Autodesk Fusion 360 part; units mm, degrees
(part 2 of 2)
sketch "Sketch5" plane through (0, 0, -2) normal (0, 0, -1) x (1, 0, 0)
  circle A0 centre (59.3355, -41.7346) radius 3
  circle A1 centre (58.8128, 16.7193) radius 3
  circle A2 centre (6.5755, -41.7346) radius 3
  circle A3 centre (6.5514, 16.7159) radius 3
  arc A4 (0, -61.8304) -> (1, -62.8304) centre (1, -61.8304) ccw
  line L0 (1, -62.8304) -> (64.3008, -62.8304)
  arc A5 (64.3008, -62.8304) -> (65.3008, -61.8304) centre (64.3008, -61.8304) ccw
  line L1 (65.3008, -61.8304) -> (65.3008, 30)
  line L2 (65.3008, 30) -> (55.2691, 40)
  line L3 (55.2691, 40) -> (10, 40)
  line L4 (10, 40) -> (0, 30)
  line L5 (0, 30) -> (0, -61.8304)
  line L6 (49.6443, -61.9222) -> (53.0574, -58.8103)
  line L7 (39.6674, -44.8986) -> (36.2543, -48.0106)
  line L8 (36.2543, -40.0106) -> (37.2428, -44.5224)
  line L9 (61.0574, -18.8103) -> (60.0689, -14.2985)
  line L10 (52.2543, -56.0106) -> (53.2428, -60.5224)
  line L11 (61.0574, -50.8103) -> (60.0689, -46.2985)
  line L12 (55.6674, -44.8986) -> (52.2543, -48.0106)
  line L13 (53.0574, -58.8103) -> (52.0689, -54.2985)
  line L14 (39.6674, -12.8986) -> (36.2543, -16.0106)
  line L15 (52.2543, -16.0106) -> (53.2428, -20.5224)
  line L16 (53.2428, -20.5224) -> (57.6443, -21.9222)
  line L17 (53.2428, -28.5224) -> (57.6443, -29.9222)
  line L18 (53.0574, -34.8103) -> (52.0689, -30.2985)
  line L19 (61.0574, -26.8103) -> (60.0689, -22.2985)
  line L20 (52.2543, -24.0106) -> (53.2428, -28.5224)
  line L21 (52.2543, -32.0106) -> (53.2428, -36.5224)
  line L22 (61.0574, -34.8103) -> (60.0689, -30.2985)
  line L23 (60.0689, -30.2985) -> (55.6674, -28.8986)
  line L24 (49.6443, -29.9222) -> (53.0574, -26.8103)
  line L25 (55.6674, -28.8986) -> (52.2543, -32.0106)
  line L26 (57.6443, -29.9222) -> (61.0574, -26.8103)
  line L27 (49.6443, -21.9222) -> (53.0574, -18.8103)
  line L28 (53.0574, -26.8103) -> (52.0689, -22.2985)
  line L29 (60.0689, -38.2985) -> (55.6674, -36.8986)
  line L30 (45.2428, -28.5224) -> (49.6443, -29.9222)
  line L31 (39.6674, -28.8986) -> (36.2543, -32.0106)
  line L32 (45.0574, -26.8103) -> (44.0689, -22.2985)
  line L33 (33.6443, -37.9222) -> (37.0574, -34.8103)
  line L34 (44.2543, -16.0106) -> (45.2428, -20.5224)
  line L35 (37.2428, -36.5224) -> (41.6443, -37.9222)
  line L36 (44.2543, -24.0106) -> (45.2428, -28.5224)
  line L37 (44.2543, -32.0106) -> (45.2428, -36.5224)
  line L38 (41.6443, -37.9222) -> (45.0574, -34.8103)
  line L39 (37.0574, -26.8103) -> (36.0689, -22.2985)
  line L40 (44.0689, -30.2985) -> (39.6674, -28.8986)
  line L41 (52.0689, -46.2985) -> (47.6674, -44.8986)
  line L42 (45.2428, -52.5224) -> (49.6443, -53.9222)
  line L43 (61.0574, -58.8103) -> (60.0689, -54.2985)
  line L44 (45.2428, -44.5224) -> (49.6443, -45.9222)
  line L45 (52.0689, -54.2985) -> (47.6674, -52.8986)
  line L46 (53.2428, -52.5224) -> (57.6443, -53.9222)
  line L47 (36.2543, -16.0106) -> (37.2428, -20.5224)
  line L48 (45.2428, -60.5224) -> (49.6443, -61.9222)
  line L49 (53.2428, -60.5224) -> (57.6443, -61.9222)
  line L50 (60.0689, -46.2985) -> (55.6674, -44.8986)
  line L51 (55.6674, -52.8986) -> (52.2543, -56.0106)
  line L52 (60.0689, -54.2985) -> (55.6674, -52.8986)
  line L53 (49.6443, -53.9222) -> (53.0574, -50.8103)
  line L54 (47.6674, -28.8986) -> (44.2543, -32.0106)
  line L55 (41.6443, -29.9222) -> (45.0574, -26.8103)
  line L56 (33.6443, -29.9222) -> (37.0574, -26.8103)
  line L57 (49.6443, -37.9222) -> (53.0574, -34.8103)
  line L58 (57.6443, -21.9222) -> (61.0574, -18.8103)
  line L59 (57.6443, -37.9222) -> (61.0574, -34.8103)
  line L60 (60.0689, -22.2985) -> (55.6674, -20.8986)
  line L61 (55.6674, -20.8986) -> (52.2543, -24.0106)
  line L62 (53.2428, -36.5224) -> (57.6443, -37.9222)
  line L63 (44.0689, -38.2985) -> (39.6674, -36.8986)
  line L64 (45.0574, -34.8103) -> (44.0689, -30.2985)
  line L65 (47.6674, -20.8986) -> (44.2543, -24.0106)
  line L66 (39.6674, -20.8986) -> (36.2543, -24.0106)
  line L67 (33.6443, -21.9222) -> (37.0574, -18.8103)
  line L68 (36.2543, -24.0106) -> (37.2428, -28.5224)
  line L69 (37.2428, -28.5224) -> (41.6443, -29.9222)
  line L70 (37.2428, -20.5224) -> (41.6443, -21.9222)
  line L71 (41.6443, -21.9222) -> (45.0574, -18.8103)
  line L72 (44.0689, -22.2985) -> (39.6674, -20.8986)
  line L73 (36.2543, -32.0106) -> (37.2428, -36.5224)
  line L74 (37.0574, -34.8103) -> (36.0689, -30.2985)
  line L75 (37.2428, -12.5224) -> (41.6443, -13.9222)
  line L76 (29.2428, -36.5224) -> (33.6443, -37.9222)
  line L77 (31.6674, -28.8986) -> (28.2543, -32.0106)
  line L78 (61.0574, 5.1897) -> (60.0689, 9.7015)
  line L79 (44.2543, -8.0106) -> (45.2428, -12.5224)
  line L80 (33.6443, 18.0778) -> (37.0574, 21.1897)
  line L81 (55.6674, 11.1014) -> (52.2543, 7.9894)
  line L82 (36.0689, -54.2985) -> (31.6674, -52.8986)
  line L83 (33.6443, 26.0778) -> (37.0574, 29.1897)
  line L84 (47.6674, -4.8986) -> (44.2543, -8.0106)
  line L85 (44.0689, -6.2985) -> (39.6674, -4.8986)
  line L86 (37.0574, 5.1897) -> (36.0689, 9.7015)
  line L87 (21.2428, -20.5224) -> (25.6443, -21.9222)
  line L88 (29.2428, -44.5224) -> (33.6443, -45.9222)
  line L89 (44.2543, -0.0106) -> (45.2428, -4.5224)
  line L90 (33.6443, -5.9222) -> (37.0574, -2.8103)
  line L91 (15.6674, 11.1014) -> (12.2543, 7.9894)
  line L92 (37.2428, 3.4776) -> (41.6443, 2.0778)
  line L93 (36.0689, 25.7015) -> (31.6674, 27.1014)
  line L94 (44.2543, 7.9894) -> (45.2428, 3.4776)
  line L95 (29.2428, -60.5224) -> (33.6443, -61.9222)
  line L96 (41.6443, -13.9222) -> (45.0574, -10.8103)
  line L97 (36.2543, 7.9894) -> (37.2428, 3.4776)
  line L98 (36.0689, -46.2985) -> (31.6674, -44.8986)
  line L99 (37.2428, -4.5224) -> (41.6443, -5.9222)
  line L100 (13.0574, 5.1897) -> (12.0689, 9.7015)
  line L101 (44.0689, -14.2985) -> (39.6674, -12.8986)
  line L102 (39.6674, 3.1014) -> (36.2543, -0.0106)
  line L103 (45.0574, -2.8103) -> (44.0689, 1.7015)
  line L104 (28.0689, -30.2985) -> (23.6674, -28.8986)
  line L105 (31.6674, 11.1014) -> (28.2543, 7.9894)
  line L106 (28.2543, -16.0106) -> (29.2428, -20.5224)
  line L107 (15.6674, -36.8986) -> (12.2543, -40.0106)
  line L108 (25.6443, -29.9222) -> (29.0574, -26.8103)
  line L109 (57.6443, 2.0778) -> (61.0574, 5.1897)
  line L110 (28.2543, -8.0106) -> (29.2428, -12.5224)
  line L111 (13.0574, -42.8103) -> (12.0689, -38.2985)
  line L112 (31.6674, 3.1014) -> (28.2543, -0.0106)
  line L113 (28.0689, -22.2985) -> (23.6674, -20.8986)
  line L114 (47.6674, 11.1014) -> (44.2543, 7.9894)
  line L115 (57.6443, -13.9222) -> (61.0574, -10.8103)
  line L116 (25.6443, -13.9222) -> (29.0574, -10.8103)
  line L117 (31.6674, -20.8986) -> (28.2543, -24.0106)
  line L118 (29.0574, -34.8103) -> (28.0689, -30.2985)
  line L119 (23.6674, -36.8986) -> (20.2543, -40.0106)
  line L120 (21.0574, -26.8103) -> (20.0689, -22.2985)
  line L121 (53.0574, -2.8103) -> (52.0689, 1.7015)
  line L122 (17.6443, -29.9222) -> (21.0574, -26.8103)
  line L123 (20.2543, -32.0106) -> (21.2428, -36.5224)
  line L124 (29.2428, 3.4776) -> (33.6443, 2.0778)
  line L125 (20.2543, 7.9894) -> (21.2428, 3.4776)
  line L126 (21.2428, -12.5224) -> (25.6443, -13.9222)
  line L127 (17.6443, -21.9222) -> (21.0574, -18.8103)
  line L128 (39.6674, 11.1014) -> (36.2543, 7.9894)
  line L129 (29.0574, -26.8103) -> (28.0689, -22.2985)
  line L130 (36.0689, -22.2985) -> (31.6674, -20.8986)
  line L131 (29.2428, -4.5224) -> (33.6443, -5.9222)
  line L132 (29.0574, 5.1897) -> (28.0689, 9.7015)
  line L133 (28.2543, -24.0106) -> (29.2428, -28.5224)
  line L134 (53.2428, -12.5224) -> (57.6443, -13.9222)
  line L135 (23.6674, 11.1014) -> (20.2543, 7.9894)
  line L136 (49.6443, -13.9222) -> (53.0574, -10.8103)
  line L137 (9.6443, -45.9222) -> (13.0574, -42.8103)
  line L138 (29.2428, -28.5224) -> (33.6443, -29.9222)
  line L139 (5.2428, -60.5224) -> (9.6443, -61.9222)
  line L140 (9.6443, -53.9222) -> (13.0574, -50.8103)
  line L141 (37.0574, -10.8103) -> (36.0689, -6.2985)
  line L142 (5.2428, -52.5224) -> (9.6443, -53.9222)
  line L143 (12.2543, -48.0106) -> (13.2428, -52.5224)
  line L144 (36.0689, -30.2985) -> (31.6674, -28.8986)
  line L145 (36.2543, -8.0106) -> (37.2428, -12.5224)
  line L146 (36.0689, 9.7015) -> (31.6674, 11.1014)
  line L147 (4.2543, -48.0106) -> (5.2428, -52.5224)
  line L148 (12.0689, -54.2985) -> (7.6674, -52.8986)
  line L149 (4.2543, -56.0106) -> (5.2428, -60.5224)
  line L150 (36.0689, -38.2985) -> (31.6674, -36.8986)
  line L151 (33.6443, 10.0778) -> (37.0574, 13.1897)
  line L152 (36.0689, -14.2985) -> (31.6674, -12.8986)
  line L153 (13.2428, -60.5224) -> (17.6443, -61.9222)
  line L154 (15.6674, -44.8986) -> (12.2543, -48.0106)
  line L155 (29.2428, -52.5224) -> (33.6443, -53.9222)
  line L156 (7.6674, -44.8986) -> (4.2543, -48.0106)
  line L157 (5.2428, -44.5224) -> (9.6443, -45.9222)
  line L158 (36.0689, -6.2985) -> (31.6674, -4.8986)
  line L159 (41.6443, 2.0778) -> (45.0574, 5.1897)
  line L160 (45.0574, -10.8103) -> (44.0689, -6.2985)
  line L161 (29.2428, -20.5224) -> (33.6443, -21.9222)
  line L162 (41.6443, -5.9222) -> (45.0574, -2.8103)
  line L163 (36.0689, 17.7015) -> (31.6674, 19.1014)
  line L164 (44.0689, 1.7015) -> (39.6674, 3.1014)
  line L165 (39.6674, -4.8986) -> (36.2543, -8.0106)
  line L166 (20.0689, -46.2985) -> (15.6674, -44.8986)
  line L167 (36.0689, 1.7015) -> (31.6674, 3.1014)
  line L168 (13.2428, -44.5224) -> (17.6443, -45.9222)
  line L169 (33.6443, -13.9222) -> (37.0574, -10.8103)
  line L170 (36.2543, -0.0106) -> (37.2428, -4.5224)
  line L171 (36.0689, 33.7015) -> (31.6674, 35.1014)
  line L172 (13.2428, -52.5224) -> (17.6443, -53.9222)
  line L173 (37.0574, -2.8103) -> (36.0689, 1.7015)
  line L174 (20.0689, -54.2985) -> (15.6674, -52.8986)
  line L175 (33.6443, 2.0778) -> (37.0574, 5.1897)
  line L176 (47.6674, 3.1014) -> (44.2543, -0.0106)
  line L177 (52.0689, -38.2985) -> (47.6674, -36.8986)
  line L178 (45.0574, -42.8103) -> (44.0689, -38.2985)
  line L179 (45.2428, -20.5224) -> (49.6443, -21.9222)
  line L180 (53.0574, -42.8103) -> (52.0689, -38.2985)
  line L181 (52.0689, -30.2985) -> (47.6674, -28.8986)
  line L182 (45.2428, -36.5224) -> (49.6443, -37.9222)
  line L183 (52.0689, -22.2985) -> (47.6674, -20.8986)
  line L184 (47.6674, -36.8986) -> (44.2543, -40.0106)
  line L185 (39.6674, -36.8986) -> (36.2543, -40.0106)
  line L186 (55.6674, -36.8986) -> (52.2543, -40.0106)
  line L187 (61.0574, -42.8103) -> (60.0689, -38.2985)
  line L188 (37.0574, -42.8103) -> (36.0689, -38.2985)
  line L189 (12.2543, -56.0106) -> (13.2428, -60.5224)
  line L190 (12.0689, -46.2985) -> (7.6674, -44.8986)
  line L191 (4.2543, -40.0106) -> (5.2428, -44.5224)
  line L192 (7.6674, -52.8986) -> (4.2543, -56.0106)
  line L193 (23.6674, -12.8986) -> (20.2543, -16.0106)
  line L194 (55.6674, -12.8986) -> (52.2543, -16.0106)
  line L195 (53.0574, -18.8103) -> (52.0689, -14.2985)
  line L196 (7.6674, -12.8986) -> (4.2543, -16.0106)
  line L197 (15.6674, -12.8986) -> (12.2543, -16.0106)
  line L198 (9.6443, -61.9222) -> (13.0574, -58.8103)
  line L199 (13.0574, -58.8103) -> (12.0689, -54.2985)
  line L200 (45.0574, -18.8103) -> (44.0689, -14.2985)
  line L201 (15.6674, -52.8986) -> (12.2543, -56.0106)
  line L202 (12.2543, -40.0106) -> (13.2428, -44.5224)
  line L203 (4.2543, -32.0106) -> (5.2428, -36.5224)
  line L204 (17.6443, -13.9222) -> (21.0574, -10.8103)
  line L205 (4.2543, -16.0106) -> (5.2428, -20.5224)
  line L206 (12.2543, -16.0106) -> (13.2428, -20.5224)
  line L207 (4.2543, -24.0106) -> (5.2428, -28.5224)
  line L208 (39.6674, 35.1014) -> (36.2543, 31.9894)
  line L209 (15.6674, -20.8986) -> (12.2543, -24.0106)
  line L210 (23.6674, -4.8986) -> (20.2543, -8.0106)
  line L211 (29.0574, -10.8103) -> (28.0689, -6.2985)
  line L212 (45.2428, -12.5224) -> (49.6443, -13.9222)
  line L213 (9.6443, -29.9222) -> (13.0574, -26.8103)
  line L214 (45.2428, -4.5224) -> (49.6443, -5.9222)
  line L215 (45.2428, 3.4776) -> (49.6443, 2.0778)
  line L216 (52.0689, -6.2985) -> (47.6674, -4.8986)
  line L217 (41.6443, 10.0778) -> (45.0574, 13.1897)
  line L218 (12.2543, -32.0106) -> (13.2428, -36.5224)
  line L219 (21.0574, -10.8103) -> (20.0689, -6.2985)
  line L220 (37.0574, 29.1897) -> (36.0689, 33.7015)
  line L221 (44.0689, 9.7015) -> (39.6674, 11.1014)
  line L222 (60.0689, -14.2985) -> (55.6674, -12.8986)
  line L223 (20.2543, -8.0106) -> (21.2428, -12.5224)
  line L224 (44.2543, 15.9894) -> (45.2428, 11.4776)
  line L225 (21.2428, -4.5224) -> (25.6443, -5.9222)
  line L226 (52.0689, 1.7015) -> (47.6674, 3.1014)
  line L227 (45.0574, 13.1897) -> (44.0689, 17.7015)
  line L228 (47.6674, 19.1014) -> (44.2543, 15.9894)
  line L229 (52.0689, -14.2985) -> (47.6674, -12.8986)
  line L230 (37.0574, 13.1897) -> (36.0689, 17.7015)
  line L231 (12.0689, -22.2985) -> (7.6674, -20.8986)
  line L232 (52.0689, 17.7015) -> (47.6674, 19.1014)
  line L233 (45.2428, 19.4776) -> (49.6443, 18.0778)
  line L234 (5.2428, 3.4776) -> (9.6443, 2.0778)
  line L235 (29.0574, -42.8103) -> (28.0689, -38.2985)
  line L236 (9.6443, -37.9222) -> (13.0574, -34.8103)
  line L237 (12.2543, 7.9894) -> (13.2428, 3.4776)
  line L238 (9.6443, -21.9222) -> (13.0574, -18.8103)
  line L239 (45.2428, 27.4776) -> (49.6443, 26.0778)
  line L240 (12.0689, 1.7015) -> (7.6674, 3.1014)
  line L241 (12.0689, -6.2985) -> (7.6674, -4.8986)
  line L242 (47.6674, 35.1014) -> (44.2543, 31.9894)
  line L243 (31.6674, -36.8986) -> (28.2543, -40.0106)
  line L244 (12.0689, -38.2985) -> (7.6674, -36.8986)
  line L245 (44.0689, 25.7015) -> (39.6674, 27.1014)
  line L246 (13.0574, -26.8103) -> (12.0689, -22.2985)
  line L247 (7.6674, -28.8986) -> (4.2543, -32.0106)
  line L248 (5.2428, -20.5224) -> (9.6443, -21.9222)
  line L249 (4.2543, -0.0106) -> (5.2428, -4.5224)
  line L250 (44.0689, 33.7015) -> (39.6674, 35.1014)
  line L251 (52.0689, 25.7015) -> (47.6674, 27.1014)
  line L252 (39.6674, 27.1014) -> (36.2543, 23.9894)
  line L253 (4.2543, -8.0106) -> (5.2428, -12.5224)
  line L254 (20.0689, -38.2985) -> (15.6674, -36.8986)
  line L255 (44.2543, 31.9894) -> (45.2428, 27.4776)
  line L256 (12.2543, -24.0106) -> (13.2428, -28.5224)
  line L257 (5.2428, -28.5224) -> (9.6443, -29.9222)
  line L258 (45.0574, 21.1897) -> (44.0689, 25.7015)
  line L259 (13.2428, -28.5224) -> (17.6443, -29.9222)
  line L260 (41.6443, 26.0778) -> (45.0574, 29.1897)
  line L261 (13.0574, -10.8103) -> (12.0689, -6.2985)
  line L262 (45.0574, 29.1897) -> (44.0689, 33.7015)
  line L263 (7.6674, -20.8986) -> (4.2543, -24.0106)
  line L264 (37.2428, 27.4776) -> (41.6443, 26.0778)
  line L265 (12.2543, -0.0106) -> (13.2428, -4.5224)
  line L266 (9.6443, -13.9222) -> (13.0574, -10.8103)
  line L267 (28.0689, -14.2985) -> (23.6674, -12.8986)
  line L268 (55.6674, -4.8986) -> (52.2543, -8.0106)
  line L269 (49.6443, 2.0778) -> (53.0574, 5.1897)
  line L270 (60.0689, 1.7015) -> (55.6674, 3.1014)
  line L271 (45.0574, 5.1897) -> (44.0689, 9.7015)
  line L272 (53.0574, 5.1897) -> (52.0689, 9.7015)
  line L273 (28.2543, -32.0106) -> (29.2428, -36.5224)
  line L274 (60.0689, -6.2985) -> (55.6674, -4.8986)
  line L275 (49.6443, -5.9222) -> (53.0574, -2.8103)
  line L276 (21.0574, -42.8103) -> (20.0689, -38.2985)
  line L277 (28.2543, 7.9894) -> (29.2428, 3.4776)
  line L278 (17.6443, -37.9222) -> (21.0574, -34.8103)
  line L279 (17.6443, 2.0778) -> (21.0574, 5.1897)
  line L280 (53.0574, -10.8103) -> (52.0689, -6.2985)
  line L281 (23.6674, 3.1014) -> (20.2543, -0.0106)
  line L282 (55.6674, 3.1014) -> (52.2543, -0.0106)
  line L283 (7.6674, -36.8986) -> (4.2543, -40.0106)
  line L284 (23.6674, -20.8986) -> (20.2543, -24.0106)
  line L285 (17.6443, -5.9222) -> (21.0574, -2.8103)
  line L286 (21.0574, 5.1897) -> (20.0689, 9.7015)
  line L287 (21.2428, -36.5224) -> (25.6443, -37.9222)
  line L288 (20.2543, -16.0106) -> (21.2428, -20.5224)
  line L289 (23.6674, -28.8986) -> (20.2543, -32.0106)
  line L290 (53.2428, -4.5224) -> (57.6443, -5.9222)
  line L291 (28.0689, -38.2985) -> (23.6674, -36.8986)
  line L292 (25.6443, 2.0778) -> (29.0574, 5.1897)
  line L293 (31.6674, -4.8986) -> (28.2543, -8.0106)
  line L294 (21.0574, -2.8103) -> (20.0689, 1.7015)
  line L295 (25.6443, -21.9222) -> (29.0574, -18.8103)
  line L296 (20.2543, -24.0106) -> (21.2428, -28.5224)
  line L297 (20.2543, -0.0106) -> (21.2428, -4.5224)
  line L298 (37.2428, 19.4776) -> (41.6443, 18.0778)
  line L299 (52.2543, 7.9894) -> (53.2428, 3.4776)
  line L300 (53.2428, 3.4776) -> (57.6443, 2.0778)
  line L301 (21.2428, 3.4776) -> (25.6443, 2.0778)
  line L302 (25.6443, -37.9222) -> (29.0574, -34.8103)
  line L303 (61.0574, -10.8103) -> (60.0689, -6.2985)
  line L304 (29.2428, -12.5224) -> (33.6443, -13.9222)
  line L305 (52.2543, -8.0106) -> (53.2428, -12.5224)
  line L306 (21.0574, -34.8103) -> (20.0689, -30.2985)
  line L307 (57.6443, -5.9222) -> (61.0574, -2.8103)
  line L308 (37.2428, 11.4776) -> (41.6443, 10.0778)
  line L309 (61.0574, -2.8103) -> (60.0689, 1.7015)
  line L310 (28.0689, 1.7015) -> (23.6674, 3.1014)
  line L311 (44.0689, 17.7015) -> (39.6674, 19.1014)
  line L312 (29.0574, -2.8103) -> (28.0689, 1.7015)
  line L313 (21.2428, -28.5224) -> (25.6443, -29.9222)
  line L314 (25.6443, -5.9222) -> (29.0574, -2.8103)
  line L315 (36.2543, 15.9894) -> (37.2428, 11.4776)
  line L316 (28.0689, -6.2985) -> (23.6674, -4.8986)
  line L317 (28.2543, -0.0106) -> (29.2428, -4.5224)
  line L318 (52.2543, -0.0106) -> (53.2428, -4.5224)
  line L319 (39.6674, 19.1014) -> (36.2543, 15.9894)
  line L320 (33.6443, -53.9222) -> (37.0574, -50.8103)
  line L321 (33.6443, -45.9222) -> (37.0574, -42.8103)
  line L322 (39.6674, -52.8986) -> (36.2543, -56.0106)
  line L323 (44.2543, -56.0106) -> (45.2428, -60.5224)
  line L324 (37.2428, -52.5224) -> (41.6443, -53.9222)
  line L325 (41.6443, -45.9222) -> (45.0574, -42.8103)
  line L326 (45.0574, -58.8103) -> (44.0689, -54.2985)
  line L327 (37.0574, -58.8103) -> (36.0689, -54.2985)
  line L328 (45.0574, -50.8103) -> (44.0689, -46.2985)
  line L329 (47.6674, -44.8986) -> (44.2543, -48.0106)
  line L330 (44.2543, -48.0106) -> (45.2428, -52.5224)
  line L331 (44.0689, -54.2985) -> (39.6674, -52.8986)
  line L332 (44.2543, -40.0106) -> (45.2428, -44.5224)
  line L333 (44.0689, -46.2985) -> (39.6674, -44.8986)
  line L334 (41.6443, -61.9222) -> (45.0574, -58.8103)
  line L335 (37.2428, -44.5224) -> (41.6443, -45.9222)
  line L336 (33.6443, -61.9222) -> (37.0574, -58.8103)
  line L337 (36.2543, -48.0106) -> (37.2428, -52.5224)
  line L338 (41.6443, -53.9222) -> (45.0574, -50.8103)
  line L339 (52.2543, -48.0106) -> (53.2428, -52.5224)
  line L340 (53.0574, -50.8103) -> (52.0689, -46.2985)
  line L341 (53.2428, -44.5224) -> (57.6443, -45.9222)
  line L342 (36.2543, -56.0106) -> (37.2428, -60.5224)
  line L343 (57.6443, -45.9222) -> (61.0574, -42.8103)
  line L344 (57.6443, -61.9222) -> (61.0574, -58.8103)
  line L345 (52.2543, -40.0106) -> (53.2428, -44.5224)
  line L346 (37.0574, -50.8103) -> (36.0689, -46.2985)
  line L347 (37.2428, -60.5224) -> (41.6443, -61.9222)
  line L348 (49.6443, -45.9222) -> (53.0574, -42.8103)
  line L349 (57.6443, -53.9222) -> (61.0574, -50.8103)
  line L350 (47.6674, -52.8986) -> (44.2543, -56.0106)
  line L351 (13.0574, -18.8103) -> (12.0689, -14.2985)
  line L352 (31.6674, -12.8986) -> (28.2543, -16.0106)
  line L353 (29.0574, -18.8103) -> (28.0689, -14.2985)
  line L354 (21.0574, -18.8103) -> (20.0689, -14.2985)
  line L355 (37.0574, -18.8103) -> (36.0689, -14.2985)
  line L356 (17.6443, -53.9222) -> (21.0574, -50.8103)
  line L357 (28.2543, -56.0106) -> (29.2428, -60.5224)
  line L358 (25.6443, -53.9222) -> (29.0574, -50.8103)
  line L359 (28.0689, -54.2985) -> (23.6674, -52.8986)
  line L360 (31.6674, -44.8986) -> (28.2543, -48.0106)
  line L361 (20.2543, -56.0106) -> (21.2428, -60.5224)
  line L362 (29.0574, -50.8103) -> (28.0689, -46.2985)
  line L363 (28.0689, -46.2985) -> (23.6674, -44.8986)
  line L364 (21.0574, -50.8103) -> (20.0689, -46.2985)
  line L365 (28.2543, -40.0106) -> (29.2428, -44.5224)
  line L366 (28.2543, -48.0106) -> (29.2428, -52.5224)
  line L367 (20.2543, -48.0106) -> (21.2428, -52.5224)
  line L368 (21.0574, -58.8103) -> (20.0689, -54.2985)
  line L369 (31.6674, -52.8986) -> (28.2543, -56.0106)
  line L370 (13.0574, -50.8103) -> (12.0689, -46.2985)
  line L371 (17.6443, -61.9222) -> (21.0574, -58.8103)
  line L372 (20.2543, -40.0106) -> (21.2428, -44.5224)
  line L373 (21.2428, -44.5224) -> (25.6443, -45.9222)
  line L374 (29.0574, -58.8103) -> (28.0689, -54.2985)
  line L375 (21.2428, -52.5224) -> (25.6443, -53.9222)
  line L376 (25.6443, -45.9222) -> (29.0574, -42.8103)
  line L377 (17.6443, -45.9222) -> (21.0574, -42.8103)
  line L378 (23.6674, -44.8986) -> (20.2543, -48.0106)
  line L379 (25.6443, -61.9222) -> (29.0574, -58.8103)
  line L380 (23.6674, -52.8986) -> (20.2543, -56.0106)
  line L381 (21.2428, -60.5224) -> (25.6443, -61.9222)
  line L382 (13.0574, -2.8103) -> (12.0689, 1.7015)
  line L383 (13.2428, -36.5224) -> (17.6443, -37.9222)
  line L384 (13.2428, -12.5224) -> (17.6443, -13.9222)
  line L385 (12.2543, -8.0106) -> (13.2428, -12.5224)
  line L386 (20.0689, -30.2985) -> (15.6674, -28.8986)
  line L387 (7.6674, 3.1014) -> (4.2543, -0.0106)
  line L388 (5.2428, -12.5224) -> (9.6443, -13.9222)
  line L389 (15.6674, 3.1014) -> (12.2543, -0.0106)
  line L390 (47.6674, 27.1014) -> (44.2543, 23.9894)
  line L391 (9.6443, 2.0778) -> (13.0574, 5.1897)
  line L392 (12.0689, -30.2985) -> (7.6674, -28.8986)
  line L393 (44.2543, 23.9894) -> (45.2428, 19.4776)
  line L394 (13.0574, -34.8103) -> (12.0689, -30.2985)
  line L395 (52.0689, 33.7015) -> (47.6674, 35.1014)
  line L396 (5.2428, -4.5224) -> (9.6443, -5.9222)
  line L397 (20.0689, 1.7015) -> (15.6674, 3.1014)
  line L398 (37.0574, 21.1897) -> (36.0689, 25.7015)
  line L399 (41.6443, 18.0778) -> (45.0574, 21.1897)
  line L400 (20.0689, 9.7015) -> (15.6674, 11.1014)
  line L401 (15.6674, -28.8986) -> (12.2543, -32.0106)
  line L402 (4.2543, 7.9894) -> (5.2428, 3.4776)
  line L403 (13.2428, -20.5224) -> (17.6443, -21.9222)
  line L404 (36.2543, 31.9894) -> (37.2428, 27.4776)
  line L405 (5.2428, -36.5224) -> (9.6443, -37.9222)
  line L406 (12.0689, -14.2985) -> (7.6674, -12.8986)
  line L407 (36.2543, 23.9894) -> (37.2428, 19.4776)
  line L408 (7.6674, 11.1014) -> (4.2543, 7.9894)
  line L409 (20.0689, -22.2985) -> (15.6674, -20.8986)
  line L410 (9.6443, -5.9222) -> (13.0574, -2.8103)
  line L411 (15.6674, -4.8986) -> (12.2543, -8.0106)
  line L412 (20.0689, -6.2985) -> (15.6674, -4.8986)
  line L413 (29.2428, 11.4776) -> (33.6443, 10.0778)
  line L414 (49.6443, 26.0778) -> (53.0574, 29.1897)
  line L415 (52.2543, 15.9894) -> (53.2428, 11.4776)
  line L416 (21.2428, 19.4776) -> (25.6443, 18.0778)
  line L417 (28.0689, 9.7015) -> (23.6674, 11.1014)
  line L418 (20.0689, 33.7015) -> (15.6674, 35.1014)
  line L419 (53.0574, 13.1897) -> (52.0689, 17.7015)
  line L420 (52.0689, 9.7015) -> (47.6674, 11.1014)
  line L421 (52.2543, 31.9894) -> (53.2428, 27.4776)
  line L422 (23.6674, 19.1014) -> (20.2543, 15.9894)
  line L423 (29.0574, 13.1897) -> (28.0689, 17.7015)
  line L424 (13.2428, 19.4776) -> (17.6443, 18.0778)
  line L425 (61.0574, 21.1897) -> (60.0689, 25.7015)
  line L426 (20.0689, 17.7015) -> (15.6674, 19.1014)
  line L427 (53.2428, 11.4776) -> (57.6443, 10.0778)
  line L428 (20.0689, 25.7015) -> (15.6674, 27.1014)
  line L429 (13.2428, 3.4776) -> (17.6443, 2.0778)
  line L430 (13.2428, 11.4776) -> (17.6443, 10.0778)
  line L431 (20.0689, -14.2985) -> (15.6674, -12.8986)
  line L432 (45.2428, 11.4776) -> (49.6443, 10.0778)
  line L433 (13.2428, -4.5224) -> (17.6443, -5.9222)
  line L434 (25.6443, 10.0778) -> (29.0574, 13.1897)
  line L435 (55.6674, 27.1014) -> (52.2543, 23.9894)
  line L436 (57.6443, 26.0778) -> (61.0574, 29.1897)
  line L437 (28.2543, 15.9894) -> (29.2428, 11.4776)
  line L438 (29.2428, 19.4776) -> (33.6443, 18.0778)
  line L439 (7.6674, -4.8986) -> (4.2543, -8.0106)
  line L440 (21.2428, 11.4776) -> (25.6443, 10.0778)
  line L441 (61.0574, 29.1897) -> (60.0689, 33.7015)
  line L442 (13.2428, 27.4776) -> (17.6443, 26.0778)
  line L443 (28.0689, 17.7015) -> (23.6674, 19.1014)
  line L444 (60.0689, 9.7015) -> (55.6674, 11.1014)
  line L445 (60.0689, 25.7015) -> (55.6674, 27.1014)
  line L446 (60.0689, 17.7015) -> (55.6674, 19.1014)
  line L447 (7.6674, 19.1014) -> (4.2543, 15.9894)
  line L448 (29.0574, 29.1897) -> (28.0689, 33.7015)
  line L449 (53.2428, 19.4776) -> (57.6443, 18.0778)
  line L450 (12.2543, 15.9894) -> (13.2428, 11.4776)
  line L451 (61.0574, 13.1897) -> (60.0689, 17.7015)
  line L452 (4.2543, 31.9894) -> (5.2428, 27.4776)
  line L453 (60.0689, 33.7015) -> (55.6674, 35.1014)
  line L454 (55.6674, 19.1014) -> (52.2543, 15.9894)
  line L455 (9.6443, 18.0778) -> (13.0574, 21.1897)
  line L456 (49.6443, 18.0778) -> (53.0574, 21.1897)
  line L457 (55.6674, 35.1014) -> (52.2543, 31.9894)
  line L458 (9.6443, 10.0778) -> (13.0574, 13.1897)
  line L459 (53.0574, 21.1897) -> (52.0689, 25.7015)
  line L460 (12.0689, 9.7015) -> (7.6674, 11.1014)
  line L461 (20.2543, 15.9894) -> (21.2428, 11.4776)
  line L462 (5.2428, 11.4776) -> (9.6443, 10.0778)
  line L463 (57.6443, 18.0778) -> (61.0574, 21.1897)
  line L464 (57.6443, 10.0778) -> (61.0574, 13.1897)
  line L465 (4.2543, 23.9894) -> (5.2428, 19.4776)
  line L466 (12.0689, 33.7015) -> (7.6674, 35.1014)
  line L467 (25.6443, 18.0778) -> (29.0574, 21.1897)
  line L468 (21.0574, 13.1897) -> (20.0689, 17.7015)
  line L469 (15.6674, 19.1014) -> (12.2543, 15.9894)
  line L470 (17.6443, 10.0778) -> (21.0574, 13.1897)
  line L471 (25.6443, 26.0778) -> (29.0574, 29.1897)
  line L472 (52.2543, 23.9894) -> (53.2428, 19.4776)
  line L473 (31.6674, 19.1014) -> (28.2543, 15.9894)
  line L474 (12.2543, 31.9894) -> (13.2428, 27.4776)
  line L475 (49.6443, 10.0778) -> (53.0574, 13.1897)
  line L476 (53.0574, 29.1897) -> (52.0689, 33.7015)
  line L477 (20.2543, 31.9894) -> (21.2428, 27.4776)
  line L478 (31.6674, 27.1014) -> (28.2543, 23.9894)
  line L479 (12.0689, 17.7015) -> (7.6674, 19.1014)
  line L480 (13.0574, 13.1897) -> (12.0689, 17.7015)
  line L481 (17.6443, 26.0778) -> (21.0574, 29.1897)
  line L482 (23.6674, 27.1014) -> (20.2543, 23.9894)
  line L483 (13.0574, 21.1897) -> (12.0689, 25.7015)
  line L484 (5.2428, 27.4776) -> (9.6443, 26.0778)
  line L485 (12.0689, 25.7015) -> (7.6674, 27.1014)
  line L486 (53.2428, 27.4776) -> (57.6443, 26.0778)
  line L487 (28.0689, 25.7015) -> (23.6674, 27.1014)
  line L488 (28.2543, 31.9894) -> (29.2428, 27.4776)
  line L489 (7.6674, 35.1014) -> (4.2543, 31.9894)
  line L490 (4.2543, 15.9894) -> (5.2428, 11.4776)
  line L491 (28.0689, 33.7015) -> (23.6674, 35.1014)
  line L492 (17.6443, 18.0778) -> (21.0574, 21.1897)
  line L493 (20.2543, 23.9894) -> (21.2428, 19.4776)
  line L494 (12.2543, 23.9894) -> (13.2428, 19.4776)
  line L495 (21.2428, 27.4776) -> (25.6443, 26.0778)
  line L496 (7.6674, 27.1014) -> (4.2543, 23.9894)
  line L497 (13.0574, 29.1897) -> (12.0689, 33.7015)
  line L498 (28.2543, 23.9894) -> (29.2428, 19.4776)
  line L499 (31.6674, 35.1014) -> (28.2543, 31.9894)
  line L500 (21.0574, 21.1897) -> (20.0689, 25.7015)
  line L501 (21.0574, 29.1897) -> (20.0689, 33.7015)
  line L502 (15.6674, 27.1014) -> (12.2543, 23.9894)
  line L503 (29.0574, 21.1897) -> (28.0689, 25.7015)
  line L504 (9.6443, 26.0778) -> (13.0574, 29.1897)
  line L505 (15.6674, 35.1014) -> (12.2543, 31.9894)
  line L506 (29.2428, 27.4776) -> (33.6443, 26.0778)
  line L507 (5.2428, 19.4776) -> (9.6443, 18.0778)
  line L508 (23.6674, 35.1014) -> (20.2543, 31.9894)
  line L509 (47.6674, -12.8986) -> (44.2543, -16.0106)
  point P0 (32.6559, -17.4104)
  point P1 (0.3608, -27.2433)
  dimension "d132" = 8
  dimension "d133" = 8
  dimension "d134" = 4
  measures "d134" distance of P0 L67
extrude "Extrude5" add sketch "Sketch5" along normal blind 0.3 contours A0 L12 L29 L50 L59 L62 L180 L186 L187 L341 L343 L345 L348 | L11 L12 L46 L50 L51 L52 L53 L339 L340 L341 L343 L349 | L17 L18 L21 L22 L23 L25 L26 L29 L57 L59 L62 L186 | L6 L10 L13 L43 L46 L49 L51 L52 L344 L349 | L12 L41 L42 L44 L45 L53 L328 L329 L330 L338 L339 L340 L348 L350 | L41 L44 L57 L177 L178 L180 L182 L184 L186 L325 L329 L332 L345 L348 | L16 L17 L19 L20 L23 L24 L25 L26 L28 L58 L60 L61 | L18 L21 L24 L25 L30 L37 L38 L54 L57 L64 L177 L181 L182 L184 | L6 L10 L13 L42 L45 L48 L51 L53 L323 L326 L334 L350 | L9 L15 L16 L27 L58 L60 L61 L115 L134 L194 L195 L222 | L20 L24 L27 L28 L30 L32 L36 L54 L55 L61 L65 L179 L181 L183 | L7 L320 L322 L324 L325 L328 L329 L330 L331 L333 L335 L337 L338 L346 | L7 L8 L35 L38 L63 L178 L184 L185 L188 L321 L325 L332 L333 L335 | L322 L323 L324 L326 L327 L331 L334 L336 L338 L342 L347 L350 | L31 L33 L35 L37 L38 L40 L54 L55 L63 L64 L69 L73 L74 L185 | L115 L134 L136 L194 L222 L268 L274 L280 L290 L303 L305 L307 | L15 L27 L34 L65 L71 L136 L179 L183 L194 L195 L200 L212 L229 L509 | L31 L32 L36 L39 L40 L55 L56 L65 L66 L68 L69 L70 L71 L72 | L109 L121 L268 L270 L274 L275 L282 L290 L300 L307 L309 L318 | L7 L82 L88 L98 L155 L320 L321 L337 L346 L358 L360 L362 L366 L369 | L8 L33 L76 L88 L98 L150 L185 L188 L235 L243 L321 L360 L365 L376 | L79 L84 L96 L136 L160 L212 L214 L216 L229 L268 L275 L280 L305 L509 | L82 L95 L155 L320 L322 L327 L336 L342 L357 L369 L374 L379 | L31 L33 L56 L73 L74 L76 L77 L118 L138 L144 L150 L243 L273 L302 | L14 L34 L47 L66 L67 L70 L71 L72 L75 L96 L101 L200 L355 L509 | L78 L81 L109 L269 L270 L272 L282 L299 L300 L427 L444 L464 | L84 L89 L103 L121 L162 L176 L214 L215 L216 L226 L269 L275 L282 L318 | L357 L358 L359 L361 L368 L369 L371 L374 L375 L379 L380 L381 | L39 L56 L66 L67 L68 L77 L108 L117 L129 L130 L133 L138 L144 L161 | L356 L358 L359 L360 L362 L363 L364 L366 L367 L373 L375 L376 L378 L380 | L119 L235 L243 L276 L287 L291 L302 L363 L365 L372 L373 L376 L377 L378 | L14 L75 L79 L84 L85 L96 L99 L101 L141 L145 L160 L162 L165 L169 | A1 L81 L415 L419 L427 L444 L449 L451 L454 L464 L475 | L77 L104 L108 L118 L119 L123 L273 L278 L287 L289 L291 L302 L306 L313 | L81 L94 L114 L159 L176 L215 L226 L269 L271 L272 L299 L420 L432 L475 | L153 L172 L174 L189 L198 L199 L201 L356 L361 L368 L371 L380 | L14 L47 L67 L106 L117 L130 L152 L161 L169 L295 L304 L352 L353 L355 | L85 L89 L90 L92 L99 L102 L103 L159 L162 L164 L165 L170 L173 L176 | L87 L104 L108 L113 L117 L120 L122 L129 L133 L284 L289 L295 L296 L313 | L114 L217 L224 L227 L228 L232 L233 L415 L419 L420 L432 L454 L456 L475 | A1 L425 L435 L436 L445 L446 L449 L454 L456 L459 L463 L472 L486 | L139 L140 L142 L148 L149 L189 L192 L198 L199 L201 | L140 L143 L154 L166 L168 L172 L174 L201 L356 L364 L367 L370 L377 L378 | L107 L111 L119 L137 L154 L166 L168 L202 L254 L276 L278 L372 L377 L383 | L90 L110 L116 L131 L141 L145 L152 L158 L165 L169 L211 L293 L304 L352 | L107 L122 L123 L218 L236 L254 L259 L278 L289 L306 L383 L386 L394 L401 | L86 L92 L94 L97 L102 L114 L128 L159 L164 L175 L217 L221 L271 L308 | L228 L232 L233 L239 L251 L258 L390 L393 L399 L414 L435 L456 L459 L472 | L87 L106 L113 L116 L126 L127 L193 L267 L284 L288 L295 L352 L353 L354 | L414 L421 L435 L436 L441 L445 L453 L457 L476 L486 | L90 L102 L112 L124 L131 L158 L167 L170 L173 L175 L293 L312 L314 L317 | L137 L140 L142 L143 L147 L148 L154 L156 L157 L190 L192 L370 | L120 L122 L127 L209 L213 L246 L256 L259 L284 L296 L386 L401 L403 L409 | L128 L151 L217 L221 L224 L227 L228 L230 L298 L308 L311 L315 L319 L399 | L110 L116 L126 L193 L204 L210 L211 L219 L223 L225 L267 L293 L314 L316 | A2 L107 L111 L137 L156 L157 L190 L191 L202 L236 L244 L283 L405 | L239 L242 L251 L255 L260 L262 L390 L395 L414 L421 L457 L476 | L203 L213 L218 L236 L244 L247 L257 L283 L392 L394 L401 L405 | L86 L97 L105 L112 L124 L128 L132 L146 L151 L167 L175 L277 L292 L413 | L80 L245 L252 L258 L260 L264 L298 L311 L319 L390 L393 L398 L399 L407 | L127 L193 L197 L204 L206 L209 L238 L288 L351 L354 L384 L403 L409 L431 | L112 L210 L225 L281 L285 L292 L294 L297 L301 L310 L312 L314 L316 L317 | L207 L209 L213 L231 L238 L246 L247 L248 L256 L257 L263 L392 | L80 L105 L146 L151 L163 L230 L315 L319 L413 L423 L434 L437 L438 L473 | L83 L208 L220 L242 L245 L250 L252 L255 L260 L262 L264 L404 | L197 L204 L210 L219 L223 L261 L266 L285 L384 L385 L411 L412 L431 L433 | L105 L125 L132 L135 L277 L279 L281 L286 L292 L301 L310 L417 L434 L440 | L80 L83 L93 L163 L252 L398 L407 L438 L467 L473 L478 L498 L503 L506 | L196 L197 L205 L206 L231 L238 L248 L263 L266 L351 L388 L406 | L83 L93 L171 L208 L220 L404 L448 L471 L478 L488 L499 L506 | L265 L279 L281 L285 L294 L297 L382 L389 L397 L410 L411 L412 L429 L433 | L135 L416 L417 L422 L423 L434 L437 L440 L443 L461 L467 L468 L470 L473 | L196 L241 L253 L261 L266 L385 L388 L396 L406 L410 L411 L439 | L448 L471 L477 L481 L482 L487 L488 L491 L495 L499 L501 L508 | L91 L100 L125 L135 L237 L279 L286 L389 L391 L397 L400 L429 L430 L470 | L416 L422 L443 L467 L471 L478 L482 L487 L492 L493 L495 L498 L500 L503 | L234 L240 L241 L249 L265 L382 L387 L389 L391 L396 L410 L439 | L418 L428 L442 L474 L477 L481 L497 L501 L502 L504 L505 L508 | L91 L400 L422 L424 L426 L430 L450 L458 L461 L468 L469 L470 L480 L492 | L91 L100 L234 L237 L240 L387 L391 L402 L408 L458 L460 L462 | L424 L426 L428 L442 L455 L469 L481 L482 L483 L492 L493 L494 L500 L502 | L452 L466 L474 L484 L485 L489 L496 L497 L504 L505 | A3 L408 L450 L455 L458 L460 L462 L469 L479 L480 L490 L507 | A3 L455 L465 L479 L483 L484 L485 L494 L496 L502 L504 L507
